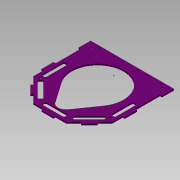
# Autodesk Inventor part: Kepala Tutup
Saved by Autodesk Inventor 2015 SP1 (Build 190203100, 203)
## iProperties
Created: 2015-02-09
Part Number: Kepala Tutup
Material: Generic
Document SubType Name: Modeling
Designer: Rafi Kurnia Putra
Density: 1 g/cm^3
Appearance: Smooth - Purple
Mass: 57.2265 g
Surface Area: 360.662 cm^2
Volume: 57.2265 cm^3
Author: Rafi Kurnia Putra
Autodesk Inventor part; units mm, degrees
ref_plane "YZ Plane" through (0, 0, 0) normal (1, 0, 0) x (0, 1, 0)
ref_plane "XZ Plane" through (0, 0, 0) normal (0, 1, 0) x (-1, 0, 0)
sketch "Sketch1" plane through (0, 0, 0) normal (0, 1, 0) x (-1, 0, 0)
  line L0 (8.7497, -92.3419) -> (8.7497, -95.2384)
  line L1 (46.7787, -69.2374) -> (48.9, -71.3587)
  line L2 (60.4053, -43.9361) -> (57.2589, -43.9361)
  line L3 (57.4053, -26.0824) -> (60.4053, -26.0824)
  line L4 (60.4053, 9.6676) -> (57.4053, 9.6675)
  line L5 (57.4053, 27.1676) -> (60.4053, 27.1676)
  line L6 (60.4053, 80.4174) -> (60.4053, 62.9175)
  line L7 (57.4053, 95.7386) -> (57.4053, 80.4174)
  line L8 (42.0845, 95.7386) -> (57.4053, 95.7386)
  line L9 (42.0845, 98.7386) -> (42.0845, 95.7386)
  line L10 (24.5845, 98.7386) -> (42.0845, 98.7386)
  line L11 (24.5845, 95.7386) -> (24.5845, 98.7386)
  line L12 (60.4053, 62.9175) -> (57.4053, 62.9175)
  line L13 (57.4053, 80.4174) -> (60.4053, 80.4174)
  arc A0 (-0.0003, -60.5669) -> (-0.0003, 14.4331) centre (-0.0003, -23.0669) ccw
  line L14 (24.5845, 95.7386) -> (-0.0003, 95.7386)
  line L15 (-0.0003, -95.2384) -> (8.7497, -95.2384)
  line L16 (8.7497, -92.3419) -> (23.6742, -92.3419)
  line L17 (23.6742, -92.3419) -> (34.4044, -81.6117)
  line L18 (48.9, -71.3587) -> (36.5257, -83.7331)
  line L19 (46.7787, -69.2374) -> (57.2589, -58.7572)
  line L20 (57.4053, 62.9175) -> (57.4053, 27.1676)
  line L21 (60.4053, 27.1676) -> (60.4053, 9.6676)
  line L22 (57.4053, 9.6675) -> (57.4053, -26.0824)
  line L23 (60.4053, -26.0824) -> (60.4053, -43.9361)
  line L24 (57.2589, -43.9361) -> (57.2589, -58.7572)
  line L25 (-0.0003, 95.7386) -> (24.5845, 95.7386)
  line L26 (8.7497, -95.2384) -> (-0.0003, -95.2384)
  line L27 (-0.0003, -95.2384) -> (-0.0003, 95.7386) construction
  line L28 (34.4044, -81.6117) -> (36.5257, -83.7331)
  line L29 (-8.7503, -92.3419) -> (-8.7503, -95.2384)
  line L30 (-60.406, 80.4174) -> (-60.406, 62.9175)
  line L31 (-57.406, 80.4174) -> (-60.406, 80.4174)
  line L32 (-57.406, 95.7386) -> (-57.406, 80.4174)
  line L33 (-42.0852, 95.7386) -> (-57.406, 95.7386)
  line L34 (-24.5852, 98.7386) -> (-42.0852, 98.7386)
  line L35 (-42.0852, 98.7386) -> (-42.0852, 95.7386)
  line L36 (-60.406, 62.9175) -> (-57.406, 62.9175)
  line L37 (-24.5852, 95.7386) -> (-24.5852, 98.7386)
  line L38 (-46.7794, -69.2374) -> (-48.9007, -71.3587)
  line L39 (-57.406, 27.1676) -> (-60.406, 27.1676)
  line L40 (-60.406, 9.6676) -> (-57.406, 9.6675)
  line L41 (-57.406, -26.0824) -> (-60.406, -26.0824)
  line L42 (-60.406, -43.9361) -> (-57.2596, -43.9361)
  arc A1 (-0.0003, 14.4331) -> (-0.0003, -60.5669) centre (-0.0003, -23.0669) ccw
  line L43 (-24.5852, 95.7386) -> (-0.0003, 95.7386)
  line L44 (-0.0003, -95.2384) -> (-8.7503, -95.2384)
  line L45 (-8.7503, -92.3419) -> (-23.6749, -92.3419)
  line L46 (-23.6749, -92.3419) -> (-34.405, -81.6117)
  line L47 (-48.9007, -71.3587) -> (-36.5264, -83.7331)
  line L48 (-46.7794, -69.2374) -> (-57.2596, -58.7572)
  line L49 (-57.406, 62.9175) -> (-57.406, 27.1676)
  line L50 (-60.406, 27.1676) -> (-60.406, 9.6676)
  line L51 (-57.406, 9.6675) -> (-57.406, -26.0824)
  line L52 (-60.406, -26.0824) -> (-60.406, -43.9361)
  line L53 (-57.2596, -43.9361) -> (-57.2596, -58.7572)
  line L54 (-8.7503, -95.2384) -> (-0.0003, -95.2384)
  line L55 (-0.0003, 95.7386) -> (-24.5852, 95.7386)
  line L56 (-34.405, -81.6117) -> (-36.5264, -83.7331)
  point P0 (-16.2126, 39.7616)
  dimension "d10" = 3
  dimension "d11" = 3
  dimension "d12" = 135
  dimension "d14" = 3
  dimension "d15" = 3
  dimension "d16" = 3
  dimension "d17" = 3
  dimension "d18" = 3
  constraints: 114 end point, 27 symmetric about line, 7 parallel, 5 vertical, 4 point on circle, 3 horizontal, 2 centre point, 2 perpendicular, 2 point on line, 2 other
  measures "d10" distance between parallel lines of L18 L19
  measures "d11" distance between parallel lines of L18 L17
  measures "d12" angle of L17 L16
  measures "d14" distance between parallel lines of L23 L22
  measures "d15" distance between parallel lines of L20 L21
  measures "d16" distance between parallel lines of L6 L7
  measures "d17" distance between parallel lines of L8 L10
  measures "d18" distance between parallel lines of L10 L14
ref_plane "Work Plane2" through (0, 3, 0) normal (0, 1, 0) x (1, 0, 0)
sketch "Sketch2" plane through (0, 3, 0) normal (0, 1, 0) x (1, 0, 0)
  circle A0 centre (-25.7175, -54.4331) radius 1.75 projected
  circle A1 centre (-25.7175, -54.4331) radius 1.75 projected
  circle A2 centre (-25.7175, -54.4331) radius 1.75 projected
  circle A3 centre (25.7175, -54.4331) radius 1.75 projected
  circle A4 centre (-25.7175, -54.4331) radius 1.75 projected
  circle A5 centre (-25.7175, -54.4331) radius 1.75 projected
  circle A6 centre (25.7175, -54.4331) radius 1.75 projected
  circle A7 centre (-49.9057, 55.0043) radius 1.75 projected
  circle A8 centre (49.906, 55.0043) radius 1.75 projected
  circle A9 centre (-50.5965, -89.4286) radius 1.75 projected
  circle A10 centre (50.5965, -89.4286) radius 1.5 projected
  circle A11 centre (-50.5965, -19.4376) radius 1.75 projected
  circle A12 centre (50.5965, -19.4376) radius 1.75 projected
  point P0 (0, 0)
extrude "Extrusion4" add sketch "Sketch1" along normal blind 2
extrude "Extrusion5" cut sketch "Sketch2" against normal through all
sketch "Sketch3" plane through (0, 2, 0) normal (0, 1, 0) x (1, 0, 0)
  line L0 (60.406, -27.1676) -> (-60.4053, -27.1676)
  line L1 (-60.4053, -27.1676) -> (-60.4053, -98.7386)
  line L2 (-60.4053, -98.7386) -> (60.406, -98.7386)
  line L3 (60.406, -98.7386) -> (60.406, -27.1676)
  circle A0 centre (44.906, -24.1676) radius 1
  circle A1 centre (44.906, -30.1676) radius 1
  circle A2 centre (23.906, -24.1676) radius 1
  circle A3 centre (23.906, -30.1676) radius 1
  line L4 (57.406, -62.9175) -> (57.406, -27.1676) projected
  line L5 (44.906, -24.1676) -> (23.906, -30.1676) construction
  line L6 (44.906, -30.1676) -> (23.906, -24.1676) construction
  line L7 (0, 0) -> (0, 20) construction
  line L8 (-60.406, -27.1676) -> (60.4053, -27.1676)
  circle A4 centre (-44.906, -24.1676) radius 1
  circle A5 centre (-44.906, -30.1676) radius 1
  circle A6 centre (-23.906, -24.1676) radius 1
  circle A7 centre (-23.906, -30.1676) radius 1
  line L9 (-44.906, -24.1676) -> (-23.906, -30.1676) construction
  line L10 (-44.906, -30.1676) -> (-23.906, -24.1676) construction
  circle A8 centre (10.5003, -24.1676) radius 1
  circle A9 centre (10.5003, -30.1676) radius 1
  circle A10 centre (-10.4997, -24.1676) radius 1
  circle A11 centre (-10.4997, -30.1676) radius 1
  point P0 (-60.4053, -27.1676)
  point P1 (-42.0845, -98.7386)
  point P2 (0.0003, -27.1676)
  dimension "d24" = 2
  dimension "d25" = 2
  dimension "d26" = 2
  dimension "d27" = 2
  dimension "d28" = 6
  dimension "d29" = 6
  dimension "d30" = 21
  dimension "d31" = 21
  dimension "d32" = 3
  dimension "d33" = 12.5
  dimension "d35" = 12.5
  dimension "d36" = 2
  dimension "d37" = 2
  dimension "d38" = 2
  dimension "d39" = 21
  dimension "d40" = 21
  dimension "d41" = 10.5
  dimension "d42" = 10.5
  constraints: 20 end point, 12 centre point, 6 symmetric about line, 2 parallel, 1 horizontal, 1 midpoint, 1 perpendicular, 1 vertical, 5 other
  measures "d24" diameter of A0
  measures "d25" diameter of A1
  measures "d26" diameter of A2
  measures "d27" diameter of A3
  measures "d28" distance of L6.start L5.start
  measures "d29" distance of L5.end L6.end
  measures "d30" distance of L5.end L6.start
  measures "d31" distance of L6.end L5.start
  measures "d32" distance from line of L0 L5.start
  measures "d33" distance from line of L6.start L4
  measures "d35" distance from line of L5.start L4
  measures "d36" diameter of A9
  measures "d37" diameter of A10
  measures "d38" diameter of A11
  measures "d39" distance of A11.centre A9.centre
  measures "d40" distance of A10.centre A8.centre
  measures "d41" horizontal distance of A11.centre point (0, -27.168)
  measures "d42" horizontal distance of A10.centre point (0, -27.168)
extrude "Extrusion6" cut sketch "Sketch3" against normal through all contours L3 L2 L1 L0 | A0 | A1 | A2 | A3 | A4 | A5 | A6 | A7 | A8 | A9 | A10 | A11
sketch "Sketch4" plane through (0, 2, 0) normal (0, 1, 0) x (1, 0, 0)
  point P0 (0, 0)
sketch "Sketch5" plane through (0, 2, 0) normal (0, 1, 0) x (1, 0, 0)
  arc A0 (7.7965, 73.9955) -> (-7.7959, 73.9955) centre (0.0003, 68.5669) ccw
  line L0 (-29.1328, 43.3526) -> (-7.7959, 73.9955)
  arc A1 (-29.1328, 43.3526) -> (0.0003, -12.4331) centre (0.0003, 23.0669) ccw
  line L1 (7.7965, 73.9955) -> (29.1335, 43.3526)
  arc A2 (0.0003, -12.4331) -> (29.1335, 43.3526) centre (0.0003, 23.0669) ccw
  line L2 (31.1733, 44.7729) -> (9.8363, 75.4158)
  arc A3 (9.8363, 75.4158) -> (-9.8356, 75.4158) centre (0.0003, 68.5669) ccw
  line L3 (-9.8356, 75.4158) -> (-31.1726, 44.7729)
  arc A4 (-31.1726, 44.7729) -> (0.0003, -14.9187) centre (0.0003, 23.0669) ccw
  arc A5 (0.0003, -14.9187) -> (31.1733, 44.7729) centre (0.0003, 23.0669) ccw
  point P0 (0, 0)
  constraints: 12 point on circle, 8 end point, 6 centre point, 17 other
extrude "Extrusion7" cut sketch "Sketch5" against normal up to next contours L1 A2 A1 L0 A0 | A5 A4 L3 A3 L2
sketch "Sketch6" plane through (0, 2, 0) normal (0, 1, 0) x (1, 0, 0)
  point P0 (0, 0)
sketch "Sketch8" plane through (0, 2, 0) normal (0, 1, 0) x (1, 0, 0)
  line L0 (-29.2779, 86.7383) -> (-51.9053, 64.1109)
  line L1 (-27.8636, 85.3241) -> (-50.4911, 62.6967)
  line L2 (50.492, 62.6967) -> (27.8646, 85.3241)
  line L3 (51.9063, 64.1109) -> (29.2788, 86.7383)
  line L4 (16.0005, 92.2384) -> (-15.9995, 92.2384)
  line L5 (16.0005, 90.2384) -> (-15.9995, 90.2384)
  line L6 (-57.4053, 50.8326) -> (-57.4053, 18.8326)
  line L7 (-55.4053, 50.8326) -> (-55.4053, 18.8326)
  line L8 (57.4063, 18.8326) -> (57.4063, 50.8326)
  line L9 (55.4063, 18.8326) -> (55.4063, 50.8326)
  line L10 (-43.3454, 57.8215) -> (-22.6874, 78.4795)
  line L11 (-22.6874, 81.3079) -> (-24.1016, 82.7221)
  line L12 (-26.9301, 82.7221) -> (-47.588, 62.0642)
  line L13 (-47.588, 59.2357) -> (-46.1738, 57.8215)
  line L14 (-14.2859, 81.7384) -> (14.4333, 81.7406)
  line L15 (14.4328, 87.7406) -> (-14.2863, 87.7384)
  line L16 (-16.2862, 85.7382) -> (-16.286, 83.7382)
  line L17 (22.9858, 78.1821) -> (43.655, 57.5129)
  line L18 (46.4834, 57.5129) -> (47.8976, 58.9271)
  line L19 (47.8976, 61.7555) -> (27.2284, 82.4248)
  line L20 (24.4, 82.4248) -> (22.9858, 81.0105)
  line L21 (-52.9042, 21.1844) -> (-52.9064, 48.8308)
  line L22 (-50.9066, 50.8309) -> (-48.9066, 50.8311)
  line L23 (-46.9064, 48.8313) -> (-46.9042, 21.1849)
  line L24 (-48.9041, 19.1847) -> (-50.9041, 19.1846)
  line L25 (52.9063, 20.5738) -> (52.9063, 49.5617)
  line L26 (50.9063, 51.5617) -> (48.9063, 51.5617)
  line L27 (46.9063, 49.5617) -> (46.9063, 20.5738)
  line L28 (48.9063, 18.5738) -> (50.9063, 18.5738)
  arc A0 (47.8976, 58.9271) -> (47.8976, 61.7555) centre (46.4834, 60.3413) ccw
  arc A1 (43.655, 57.5129) -> (46.4834, 57.5129) centre (45.0692, 58.9271) ccw
  arc A2 (22.9858, 81.0105) -> (22.9858, 78.1821) centre (24.4, 79.5963) ccw
  arc A3 (27.2284, 82.4248) -> (24.4, 82.4248) centre (25.8142, 81.0105) ccw
  arc A4 (52.9063, 49.5617) -> (50.9063, 51.5617) centre (50.9063, 49.5617) ccw
  arc A5 (48.9063, 51.5617) -> (46.9063, 49.5617) centre (48.9063, 49.5617) ccw
  arc A6 (46.9063, 20.5738) -> (48.9063, 18.5738) centre (48.9063, 20.5738) ccw
  arc A7 (50.9063, 18.5738) -> (52.9063, 20.5738) centre (50.9063, 20.5738) ccw
  arc A8 (-14.2863, 87.7384) -> (-16.2862, 85.7382) centre (-14.2862, 85.7384) ccw
  arc A9 (-16.286, 83.7382) -> (-14.2859, 81.7384) centre (-14.286, 83.7384) ccw
  arc A10 (-24.1016, 82.7221) -> (-26.9301, 82.7221) centre (-25.5159, 81.3079) ccw
  arc A11 (-22.6874, 78.4795) -> (-22.6874, 81.3079) centre (-24.1016, 79.8937) ccw
  arc A12 (-47.588, 62.0642) -> (-47.588, 59.2357) centre (-46.1738, 60.6499) ccw
  arc A13 (-46.1738, 57.8215) -> (-43.3454, 57.8215) centre (-44.7596, 59.2357) ccw
  arc A14 (-50.9066, 50.8309) -> (-52.9064, 48.8308) centre (-50.9064, 48.8309) ccw
  arc A15 (-46.9064, 48.8313) -> (-48.9066, 50.8311) centre (-48.9064, 48.8311) ccw
  arc A16 (-48.9041, 19.1847) -> (-46.9042, 21.1849) centre (-48.9042, 21.1847) ccw
  arc A17 (-52.9042, 21.1844) -> (-50.9041, 19.1846) centre (-50.9042, 21.1846) ccw
  line L29 (16.433, 85.7408) -> (16.4332, 83.7408)
  arc A18 (16.433, 85.7408) -> (14.4328, 87.7406) centre (14.433, 85.7406) ccw
  arc A19 (14.4333, 81.7406) -> (16.4332, 83.7408) centre (14.4332, 83.7406) ccw
  line L30 (57.2596, 43.9361) -> (57.2596, 58.7572) projected
  point P0 (0, 0)
  point P1 (0.0444, 85.2384)
  point P2 (16.4328, 87.7408)
  dimension "d54" = 5
  dimension "d68" = 2
  dimension "d71" = 2
  dimension "d74" = 6
  dimension "d76" = 6
  dimension "d77" = 6
  dimension "d78" = 6
  dimension "d79" = 6
  dimension "d80" = 4.353
  constraints: 60 end point, 40 point on circle, 40 tangent, 20 centre point, 18 equal radius, 10 parallel, 5 perpendicular, 5 vertical, 2 horizontal, 2 point on line, 27 other
  measures "d54" distance from line of point (0.044, 85.238) L5
  measures "d68" radius of A0
  measures "d71" radius of A18
  measures "d74" distance between parallel lines of L15 L14
  measures "d76" distance between parallel lines of L19 L17
  measures "d77" distance between parallel lines of L10 L12
  measures "d78" distance between parallel lines of L23 L21
  measures "d79" distance between parallel lines of L27 L25
extrude "Extrusion9" cut sketch "Sketch8" against normal through all
sketch "Sketch9" plane through (0, 2, 0) normal (0, 1, 0) x (1, 0, 0)
  arc A0 (-26.9301, 82.7221) -> (-24.1016, 82.7221) centre (-25.5159, 81.3079) ccw projected
  line L0 (-24.1016, 82.7221) -> (-22.6874, 81.3079) projected
  arc A1 (-22.6874, 81.3079) -> (-22.6874, 78.4795) centre (-24.1016, 79.8937) ccw projected
  line L1 (-22.6874, 78.4795) -> (-43.3454, 57.8215) projected
  arc A2 (-43.3454, 57.8215) -> (-46.1738, 57.8215) centre (-44.7596, 59.2357) ccw projected
  line L2 (-46.1738, 57.8215) -> (-47.588, 59.2357) projected
  arc A3 (-47.588, 59.2357) -> (-47.588, 62.0642) centre (-46.1738, 60.6499) ccw projected
  line L3 (-47.588, 62.0642) -> (-26.9301, 82.7221) projected
  arc A4 (-14.2859, 81.7384) -> (-16.286, 83.7382) centre (-14.286, 83.7384) ccw projected
  line L4 (-16.286, 83.7382) -> (-16.2862, 85.7382) projected
  arc A5 (-16.2862, 85.7382) -> (-14.2863, 87.7384) centre (-14.2862, 85.7384) ccw projected
  line L5 (-14.2863, 87.7384) -> (14.4328, 87.7406) projected
  arc A6 (14.4328, 87.7406) -> (16.433, 85.7408) centre (14.433, 85.7406) ccw projected
  line L6 (16.433, 85.7408) -> (16.4332, 83.7408) projected
  arc A7 (16.4332, 83.7408) -> (14.4333, 81.7406) centre (14.4332, 83.7406) ccw projected
  line L7 (14.4333, 81.7406) -> (-14.2859, 81.7384) projected
  arc A8 (-52.9064, 48.8308) -> (-50.9066, 50.8309) centre (-50.9064, 48.8309) ccw projected
  line L8 (-50.9066, 50.8309) -> (-48.9066, 50.8311) projected
  arc A9 (-48.9066, 50.8311) -> (-46.9064, 48.8313) centre (-48.9064, 48.8311) ccw projected
  line L9 (-46.9064, 48.8313) -> (-46.9042, 21.1849) projected
  arc A10 (-46.9042, 21.1849) -> (-48.9041, 19.1847) centre (-48.9042, 21.1847) ccw projected
  line L10 (-48.9041, 19.1847) -> (-50.9041, 19.1846) projected
  arc A11 (-50.9041, 19.1846) -> (-52.9042, 21.1844) centre (-50.9042, 21.1846) ccw projected
  line L11 (-52.9042, 21.1844) -> (-52.9064, 48.8308) projected
  arc A12 (50.9063, 51.5617) -> (52.9063, 49.5617) centre (50.9063, 49.5617) ccw projected
  line L12 (52.9063, 49.5617) -> (52.9063, 20.5738) projected
  arc A13 (52.9063, 20.5738) -> (50.9063, 18.5738) centre (50.9063, 20.5738) ccw projected
  line L13 (50.9063, 18.5738) -> (48.9063, 18.5738) projected
  arc A14 (48.9063, 18.5738) -> (46.9063, 20.5738) centre (48.9063, 20.5738) ccw projected
  line L14 (46.9063, 20.5738) -> (46.9063, 49.5617) projected
  arc A15 (46.9063, 49.5617) -> (48.9063, 51.5617) centre (48.9063, 49.5617) ccw projected
  line L15 (48.9063, 51.5617) -> (50.9063, 51.5617) projected
  arc A16 (47.8976, 61.7555) -> (47.8976, 58.9271) centre (46.4834, 60.3413) ccw projected
  line L16 (47.8976, 58.9271) -> (46.4834, 57.5129) projected
  arc A17 (46.4834, 57.5129) -> (43.655, 57.5129) centre (45.0692, 58.9271) ccw projected
  line L17 (43.655, 57.5129) -> (22.9858, 78.1821) projected
  arc A18 (22.9858, 78.1821) -> (22.9858, 81.0105) centre (24.4, 79.5963) ccw projected
  line L18 (22.9858, 81.0105) -> (24.4, 82.4248) projected
  arc A19 (24.4, 82.4248) -> (27.2284, 82.4248) centre (25.8142, 81.0105) ccw projected
  line L19 (27.2284, 82.4248) -> (47.8976, 61.7555) projected
  arc A20 (-9.8356, 75.4158) -> (9.8363, 75.4158) centre (0.0003, 68.5669) ccw projected
  line L20 (9.8363, 75.4158) -> (31.1733, 44.7729) projected
  arc A21 (31.1733, 44.7729) -> (-31.1726, 44.7729) centre (0.0003, 23.0669) ccw projected
  line L21 (-31.1726, 44.7729) -> (-9.8356, 75.4158) projected
  line L22 (-57.4053, -27.1676) -> (57.406, -27.1676) projected
  line L23 (57.406, -27.1676) -> (57.406, -27.1676)
  line L24 (57.406, -27.1676) -> (60.406, -27.1676) projected
  line L25 (60.406, -27.1676) -> (60.406, -9.6676) projected
  line L26 (60.406, -9.6676) -> (57.406, -9.6675) projected
  line L27 (57.406, -9.6675) -> (57.406, 26.0824) projected
  line L28 (57.406, 26.0824) -> (60.406, 26.0824) projected
  line L29 (60.406, 26.0824) -> (60.406, 43.9361) projected
  line L30 (60.406, 43.9361) -> (57.2596, 43.9361) projected
  line L31 (57.2596, 43.9361) -> (57.2596, 58.7572) projected
  line L32 (57.2596, 58.7572) -> (46.7794, 69.2374) projected
  line L33 (46.7794, 69.2374) -> (48.9007, 71.3587) projected
  line L34 (48.9007, 71.3587) -> (36.5264, 83.7331) projected
  line L35 (36.5264, 83.7331) -> (34.405, 81.6117) projected
  line L36 (34.405, 81.6117) -> (23.6749, 92.3419) projected
  line L37 (23.6749, 92.3419) -> (8.7503, 92.3419) projected
  line L38 (8.7503, 92.3419) -> (8.7503, 95.2384) projected
  line L39 (8.7503, 95.2384) -> (-8.7497, 95.2384) projected
  line L40 (-8.7497, 95.2384) -> (-8.7497, 92.3419) projected
  line L41 (-8.7497, 92.3419) -> (-23.6742, 92.3419) projected
  line L42 (-23.6742, 92.3419) -> (-34.4044, 81.6117) projected
  line L43 (-34.4044, 81.6117) -> (-36.5257, 83.7331) projected
  line L44 (-36.5257, 83.7331) -> (-48.9, 71.3587) projected
  line L45 (-48.9, 71.3587) -> (-46.7787, 69.2374) projected
  line L46 (-46.7787, 69.2374) -> (-57.2589, 58.7572) projected
  line L47 (-57.2589, 58.7572) -> (-57.2589, 43.9361) projected
  line L48 (-57.2589, 43.9361) -> (-60.4053, 43.9361) projected
  line L49 (-60.4053, 43.9361) -> (-60.4053, 26.0824) projected
  line L50 (-60.4053, 26.0824) -> (-57.4053, 26.0824) projected
  line L51 (-57.4053, 26.0824) -> (-57.4053, -9.6675) projected
  line L52 (-57.4053, -9.6675) -> (-60.4053, -9.6676) projected
  line L53 (-60.4053, -9.6676) -> (-60.4053, -27.1676) projected
  line L54 (-60.4053, -27.1676) -> (-57.4053, -27.1676) projected
  line L55 (-57.4053, -27.1676) -> (-57.4053, -27.1676) projected
  circle A22 centre (-10.4997, -24.1676) radius 1 projected
  circle A23 centre (-44.906, -24.1676) radius 1 projected
  circle A24 centre (23.906, -24.1676) radius 1 projected
  circle A25 centre (44.906, -24.1676) radius 1 projected
  circle A26 centre (-23.906, -24.1676) radius 1 projected
  circle A27 centre (10.5003, -24.1676) radius 1 projected
  circle A28 centre (-50.5965, -19.4376) radius 1.75 projected
  circle A29 centre (49.906, 55.0043) radius 1.75 projected
  circle A30 centre (-49.9057, 55.0043) radius 1.75 projected
  circle A31 centre (50.5965, -19.4376) radius 1.75 projected
  line L56 (-57.2377, -27) -> (-57.2377, -27)
  line L57 (-60.2377, -27.1676) -> (-60.2377, -9.8351)
  line L58 (-60.2377, -9.8351) -> (-57.2377, -9.8351)
  line L59 (-57.2377, -9.8351) -> (-57.2377, 26.25)
  line L60 (-57.2377, 26.25) -> (-60.2377, 26.25)
  line L61 (-60.2377, 26.25) -> (-60.2377, 43.7686)
  line L62 (-60.2377, 43.7686) -> (-57.0913, 43.7686)
  line L63 (-57.0913, 43.7686) -> (-57.0913, 58.6878)
  line L64 (-57.0913, 58.6878) -> (-46.5417, 69.2374)
  line L65 (-46.5417, 69.2374) -> (-48.663, 71.3587)
  line L66 (-48.663, 71.3587) -> (-36.5257, 83.4961)
  line L67 (-36.5257, 83.4961) -> (-34.4044, 81.3747)
  line L68 (-34.4044, 81.3747) -> (-23.6048, 92.1743)
  line L69 (-23.6048, 92.1743) -> (-8.5821, 92.1743)
  line L70 (-8.5821, 92.1743) -> (-8.5821, 95.0708)
  line L71 (-8.5821, 95.0708) -> (8.5828, 95.0708)
  line L72 (8.5828, 95.0708) -> (8.5828, 92.1743)
  line L73 (8.5828, 92.1743) -> (23.6055, 92.1743)
  line L74 (23.6055, 92.1743) -> (34.405, 81.3747)
  line L75 (34.405, 81.3747) -> (36.5264, 83.4961)
  line L76 (36.5264, 83.4961) -> (48.6637, 71.3587)
  line L77 (48.6637, 71.3587) -> (46.5424, 69.2374)
  line L78 (46.5424, 69.2374) -> (57.092, 58.6878)
  line L79 (57.092, 58.6878) -> (57.092, 43.7686)
  line L80 (57.092, 43.7686) -> (60.2384, 43.7686)
  line L81 (60.2384, 43.7686) -> (60.2384, 26.25)
  line L82 (60.2384, 26.25) -> (57.2384, 26.25)
  line L83 (57.2384, 26.25) -> (57.2384, -9.8351)
  line L84 (57.2384, -9.8351) -> (60.2384, -9.8351)
  line L85 (60.2384, -9.8351) -> (60.2384, -27.1676)
  line L86 (57.2384, -27) -> (57.2384, -27)
  point P0 (0, 0)
  dimension "d68" = 2
  dimension "d71" = 2
  dimension "d74" = 6
  dimension "d76" = 6
  dimension "d77" = 6
  dimension "d78" = 6
  dimension "d79" = 6
  dimension "d80" = 4.353
  constraints: 64 end point, 32 centre point, 2 point on line, 26 other
extrude "Extrusion10" cut sketch "Sketch9" against normal through all contours L54 L53 L52 L51 L50 L49 L48 L47 L46 L45 L44 L43 L42 L41 L40 L39 L38 L37 L36 L35 L34 L33 L32 L31 L30 L29 L28 L27 L26 L25 L24 L85 L84 L83 L82 L81 L80 L79 L78 L77 L76 L75 L74 L73 L72 L71 L70 L69 L68 L67 L66 L65 L64 L63 L62 L61 L60 L59 L58 L57
sketch "Sketch10" plane through (0, 2, 0) normal (0, 1, 0) x (1, 0, 0)
  arc A0 (-31.1726, 44.7729) -> (31.1733, 44.7729) centre (0.0003, 23.0669) ccw projected
  line L0 (9.8363, 75.4158) -> (31.1733, 44.7729) projected
  arc A1 (9.8363, 75.4158) -> (-9.8356, 75.4158) centre (0.0003, 68.5669) ccw projected
  line L1 (-31.1726, 44.7729) -> (-9.8356, 75.4158) projected
  arc A2 (-30.7146, 44.454) -> (30.7152, 44.454) centre (0.0003, 23.0669) ccw
  line L2 (-30.7146, 44.454) -> (-9.3776, 75.0969)
  arc A3 (9.3783, 75.0969) -> (-9.3776, 75.0969) centre (0.0003, 68.5669) ccw
  line L3 (9.3783, 75.0969) -> (30.7152, 44.454)
  point P0 (0, 0)
  dimension "d84" = 0.5581
  constraints: 4 end point, 4 point on circle, 2 centre point, 3 other
  measures "d84" radial gap between concentric circles of A0 A2
extrude "Extrusion11" add sketch "Sketch10" against normal blind 2
equation "\"d35\" = d33"
equation "\"d40\" = d39"
equation "\"d41\" = 0.5 * d39"
equation "\"d42\" = d41"
body "Solid2"
